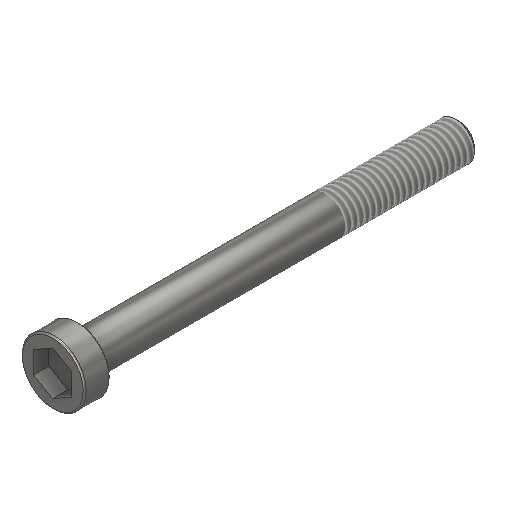
# Autodesk Inventor part: COTS_GENERIC_M5x50_Screw
Saved by Autodesk Inventor 2025 (Build 290162010, 162A)
## iProperties
Created: 2018-07-31
Part Number: COTS_GENERIC_M5x50_Screw
Material: Steel, Carbon
Document SubType Name: Modeling
Designer: Andrzej
Density: 7.85 g/cm^3
Appearance: Semi-Polished
Author: Andrzej
Autodesk Inventor part; units mm, degrees
ref_plane "YZ Plane" through (0, 0, 0) normal (1, 0, 0) x (0, 1, 0)
ref_plane "XZ Plane" through (0, 0, 0) normal (0, 1, 0) x (-1, 0, 0)
ref_plane "XY Plane" through (0, 0, 0) normal (0, 0, 1) x (1, 0, 0)
sketch "Sketch1" plane through (0, 0, 0) normal (0, 0, 1) x (1, 0, 0)
  circle A0 centre (0, 0) radius 4.2
  circle A1 centre (0, 0) radius 2.5
  dimension "d0" = 8.4
  dimension "d3" = 5
  constraints: 2 centre point, 2 coincident
  measures "d0" diameter of A0
  measures "d3" diameter of A1
extrude "Extrusion1" add sketch "Sketch1" along normal blind 3.4 contours A0 | A1
extrude "Extrusion2" add sketch "Sketch1" against normal blind 50 contours A1
thread "Thread1" size "M5x0.8" class "6g" standard "ANSI Metric M Profile" length 17.5
fillet "Fillet1" radius 0.2 2 edges at (-4.2, 0, 3.4) (-4.2, 0, 0)
chamfer "Chamfer1" distance 0.5 angle 45 1 edges at (-2.5, 0, -50)
sketch "Sketch2" plane through (0, 0, 3.4) normal (0, 0, 1) x (1, 0, 0)
  line L0 (-2.5, 1.4593) -> (0.0138, 2.8947)
  line L1 (0.0138, 2.8947) -> (2.5138, 1.4354)
  line L2 (2.5138, 1.4354) -> (2.5, -1.4593)
  line L3 (2.5, -1.4593) -> (-0.0138, -2.8947)
  line L4 (-0.0138, -2.8947) -> (-2.5138, -1.4354)
  line L5 (-2.5138, -1.4354) -> (-2.5, 1.4593)
  point P0 (0, 0)
  point P1 (0, 0)
  constraints: 12 end point, 1 coincident, 13 other
extrude "Extrusion3" cut sketch "Sketch2" against normal blind 2
body "Solid1"
